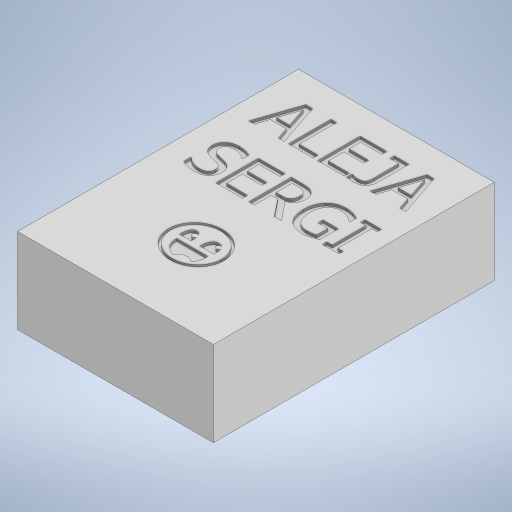
# Autodesk Inventor part: torta20personas
Saved by Autodesk Inventor 2024 (Build 280153000, 153)
## iProperties
Created: 2023-09-01
Part Number: torta20personas
Material: Genérico
Document SubType Name: Modeling
Designer: profe
Density: 1 g/cm^3
Appearance: Valor por defecto
Author: profe
Autodesk Inventor part; units mm, degrees
note: some values were not read from the file. Chosen so that the rebuilt part matches the saved one: offset side; direction of "Repujado1".
ref_plane "YZ Plane" through (0, 0, 0) normal (1, 0, 0) x (0, 1, 0)
ref_plane "XZ Plane" through (0, 0, 0) normal (0, 1, 0) x (-1, 0, 0)
ref_plane "XY Plane" through (0, 0, 0) normal (0, 0, 1) x (1, 0, 0)
sketch "Boceto2" plane through (0, 0, 0) normal (0, 1, 0) x (-1, 0, 0)
  line L0 (-115, -165) -> (115, -165)
  line L1 (115, -165) -> (115, 165)
  line L2 (115, 165) -> (-115, 165)
  line L3 (-115, 165) -> (-115, -165)
  line L4 (-115, -165) -> (115, 165) construction
  line L5 (115, -165) -> (-115, 165) construction
  point P0 (0, 0)
  dimension "d3" = 330
  dimension "d4" = 230
  constraints: 12 end point, 2 midpoint, 2 parallel, 1 horizontal, 1 perpendicular
  measures "d3" distance of L0.end L1.end
  measures "d4" distance of L0.start L0.end
extrude "Extrusión2" add sketch "Boceto2" along normal blind 100
sketch "Boceto3" plane through (0, 100, 0) normal (0, 1, 0) x (1, 0, 0)
  line L0 (-91.3257, 133.12) -> (-76.7106, 133.12) construction
  line L1 (-76.7106, 133.12) -> (-76.7106, 124.9893) construction
  line L2 (-76.7106, 124.9893) -> (-91.3257, 124.9893) construction
  line L3 (-91.3257, 124.9893) -> (-91.3257, 133.12) construction
  line L4 (-91.6498, 83.12) -> (-74.7941, 133.12)
  line L5 (-74.7941, 133.12) -> (-66.6093, 133.12)
  line L6 (-66.6093, 133.12) -> (-49.7536, 83.12)
  line L7 (-49.7536, 83.12) -> (-56.7633, 83.12)
  line L8 (-56.7633, 83.12) -> (-61.3014, 97.0989)
  line L9 (-61.3014, 97.0989) -> (-80.3857, 97.0989)
  line L10 (-80.3857, 97.0989) -> (-84.9237, 83.12)
  line L11 (-84.9237, 83.12) -> (-91.6498, 83.12)
  line L12 (-63.1247, 102.7716) -> (-70.8638, 126.3129)
  line L13 (-70.8638, 126.3129) -> (-78.5623, 102.7716)
  line L14 (-78.5623, 102.7716) -> (-63.1247, 102.7716)
  line L15 (-16.0421, 83.12) -> (-45.0129, 83.12)
  line L16 (-45.0129, 83.12) -> (-45.0129, 133.12)
  line L17 (-45.0129, 133.12) -> (-38.3678, 133.12)
  line L18 (-38.3678, 133.12) -> (-38.3678, 89.0357)
  line L19 (-38.3678, 89.0357) -> (-16.0421, 89.0357)
  line L20 (-16.0421, 89.0357) -> (-16.0421, 83.12)
  line L21 (-10.8152, 83.12) -> (-10.8152, 133.12)
  line L22 (-10.8152, 133.12) -> (20.4652, 133.12)
  line L23 (20.4652, 133.12) -> (20.4652, 127.2043)
  line L24 (20.4652, 127.2043) -> (-4.1701, 127.2043)
  line L25 (-4.1701, 127.2043) -> (-4.1701, 113.509)
  line L26 (-4.1701, 113.509) -> (18.804, 113.509)
  line L27 (18.804, 113.509) -> (18.804, 107.5933)
  line L28 (18.804, 107.5933) -> (-4.1701, 107.5933)
  line L29 (-4.1701, 107.5933) -> (-4.1701, 89.0357)
  line L30 (-4.1701, 89.0357) -> (20.4652, 89.0357)
  line L31 (20.4652, 89.0357) -> (20.4652, 83.12)
  line L32 (20.4652, 83.12) -> (-10.8152, 83.12)
  spline S0 degree 2 poles (46.5998, 96.1265) (46.5998, 89.5625) (38.5771, 82.4312) (31.8104, 82.4312) knots 0 0 0 1 2 2 2
  spline S1 degree 2 poles (31.8104, 82.4312) (30.1897, 82.4312) (24.8007, 82.9985) (22.9774, 83.4036) knots 0 0 0 1 2 2 2
  line L33 (22.9774, 83.4036) -> (22.9774, 89.8056)
  line L34 (22.9774, 89.8056) -> (23.3421, 89.8056)
  spline S2 degree 2 poles (23.3421, 89.8056) (24.7197, 89.3194) (28.8121, 88.1848) (30.919, 88.1848) knots 0 0 0 1 2 2 2
  spline S3 degree 2 poles (30.919, 88.1848) (33.9985, 88.1848) (37.6857, 89.603) (38.5365, 90.8996) knots 0 0 0 1 2 2 2
  spline S4 degree 2 poles (38.5365, 90.8996) (39.4685, 92.2367) (39.9547, 96.1265) (39.9547, 98.6792) knots 0 0 0 1 2 2 2
  line L35 (39.9547, 98.6792) -> (39.9547, 127.8121)
  line L36 (39.9547, 127.8121) -> (29.3793, 127.8121)
  line L37 (29.3793, 127.8121) -> (29.3793, 133.12)
  line L38 (29.3793, 133.12) -> (46.5998, 133.12)
  line L39 (46.5998, 133.12) -> (46.5998, 96.1265)
  line L40 (51.0163, 83.12) -> (67.872, 133.12)
  line L41 (67.872, 133.12) -> (76.0568, 133.12)
  line L42 (76.0568, 133.12) -> (92.9126, 83.12)
  line L43 (92.9126, 83.12) -> (85.9028, 83.12)
  line L44 (85.9028, 83.12) -> (81.3647, 97.0989)
  line L45 (81.3647, 97.0989) -> (62.2805, 97.0989)
  line L46 (62.2805, 97.0989) -> (57.7424, 83.12)
  line L47 (57.7424, 83.12) -> (51.0163, 83.12)
  line L48 (79.5414, 102.7716) -> (71.8023, 126.3129)
  line L49 (71.8023, 126.3129) -> (64.1038, 102.7716)
  line L50 (64.1038, 102.7716) -> (79.5414, 102.7716)
  spline S5 degree 2 poles (-72.3225, -0.0951) (-77.7519, -0.0951) (-85.3695, 2.174) (-88.7325, 3.7947) knots 0 0 0 1 2 2 2
  line L51 (-88.7325, 3.7947) -> (-88.7325, 12.1415)
  line L52 (-88.7325, 12.1415) -> (-88.2463, 12.1415)
  spline S6 degree 2 poles (-88.2463, 12.1415) (-84.9643, 9.0621) (-76.6579, 5.6586) (-72.8087, 5.6586) knots 0 0 0 1 2 2 2
  spline S7 degree 2 poles (-72.8087, 5.6586) (-67.2981, 5.6586) (-61.666, 10.2372) (-61.666, 14.0054) knots 0 0 0 1 2 2 2
  spline S8 degree 2 poles (-61.666, 14.0054) (-61.666, 17.0038) (-64.6239, 20.7315) (-67.8249, 21.6634) knots 0 0 0 1 2 2 2
  spline S9 degree 2 poles (-67.8249, 21.6634) (-70.1344, 22.3117) (-73.9837, 23.2031) (-76.8605, 23.9325) knots 0 0 0 1 2 2 2
  spline S10 degree 2 poles (-76.8605, 23.9325) (-79.4537, 24.6213) (-83.5461, 26.6877) (-85.1263, 28.349) knots 0 0 0 1 2 2 2
  spline S11 degree 2 poles (-85.1263, 28.349) (-86.666, 30.0103) (-88.3678, 34.4673) (-88.3678, 37.3847) knots 0 0 0 1 2 2 2
  spline S12 degree 2 poles (-88.3678, 37.3847) (-88.3678, 43.4625) (-78.8865, 51.6877) (-71.5526, 51.6877) knots 0 0 0 1 2 2 2
  spline S13 degree 2 poles (-71.5526, 51.6877) (-67.3387, 51.6877) (-59.8832, 50.0265) (-56.6823, 48.4462) knots 0 0 0 1 2 2 2
  line L53 (-56.6823, 48.4462) -> (-56.6823, 40.5046)
  line L54 (-56.6823, 40.5046) -> (-57.1685, 40.5046)
  spline S14 degree 2 poles (-57.1685, 40.5046) (-59.5591, 42.6926) (-67.0145, 45.9341) (-71.1069, 45.9341) knots 0 0 0 1 2 2 2
  spline S15 degree 2 poles (-71.1069, 45.9341) (-75.726, 45.9341) (-81.4391, 41.5986) (-81.4391, 38.0735) knots 0 0 0 1 2 2 2
  spline S16 degree 2 poles (-81.4391, 38.0735) (-81.4391, 34.913) (-78.0761, 31.1448) (-74.9156, 30.2939) knots 0 0 0 1 2 2 2
  spline S17 degree 2 poles (-74.9156, 30.2939) (-72.8087, 29.7266) (-66.6904, 28.268) (-64.6644, 27.6602) knots 0 0 0 1 2 2 2
  spline S18 degree 2 poles (-64.6644, 27.6602) (-59.5186, 26.08) (-54.7374, 19.7185) (-54.7374, 15.0589) knots 0 0 0 1 2 2 2
  spline S19 degree 2 poles (-54.7374, 15.0589) (-54.7374, 12.101) (-57.128, 6.4284) (-59.2754, 4.443) knots 0 0 0 1 2 2 2
  spline S20 degree 2 poles (-59.2754, 4.443) (-61.666, 2.255) (-67.7438, -0.0951) (-72.3225, -0.0951) knots 0 0 0 1 2 2 2
  line L55 (-47.9707, 0.7963) -> (-47.9707, 50.7963)
  line L56 (-47.9707, 50.7963) -> (-16.6904, 50.7963)
  line L57 (-16.6904, 50.7963) -> (-16.6904, 44.8806)
  line L58 (-16.6904, 44.8806) -> (-41.3257, 44.8806)
  line L59 (-41.3257, 44.8806) -> (-41.3257, 31.1853)
  line L60 (-41.3257, 31.1853) -> (-18.3516, 31.1853)
  line L61 (-18.3516, 31.1853) -> (-18.3516, 25.2696)
  line L62 (-18.3516, 25.2696) -> (-41.3257, 25.2696)
  line L63 (-41.3257, 25.2696) -> (-41.3257, 6.712)
  line L64 (-41.3257, 6.712) -> (-16.6904, 6.712)
  line L65 (-16.6904, 6.712) -> (-16.6904, 0.7963)
  line L66 (-16.6904, 0.7963) -> (-47.9707, 0.7963)
  line L67 (29.2983, 0.7963) -> (20.6678, 0.7963)
  line L68 (20.6678, 0.7963) -> (4.8656, 20.691)
  line L69 (4.8656, 20.691) -> (-2.7519, 20.691)
  line L70 (-2.7519, 20.691) -> (-2.7519, 0.7963)
  line L71 (-2.7519, 0.7963) -> (-9.397, 0.7963)
  line L72 (-9.397, 0.7963) -> (-9.397, 50.7963)
  line L73 (-9.397, 50.7963) -> (3.4879, 50.7963)
  spline S21 degree 2 poles (3.4879, 50.7963) (7.7829, 50.7963) (13.5771, 49.8644) (16.2108, 48.1626) knots 0 0 0 1 2 2 2
  spline S22 degree 2 poles (16.2108, 48.1626) (18.8445, 46.4608) (21.8834, 41.1529) (21.8834, 37.2226) knots 0 0 0 1 2 2 2
  spline S23 degree 2 poles (21.8834, 37.2226) (21.8834, 31.7526) (16.2918, 24.3377) (11.5106, 22.5548) knots 0 0 0 1 2 2 2
  line L74 (11.5106, 22.5548) -> (29.2983, 0.7963)
  spline S24 degree 2 poles (14.9547, 36.6958) (14.9547, 38.8838) (13.415, 42.2469) (11.7942, 43.3409) knots 0 0 0 1 2 2 2
  spline S25 degree 2 poles (11.7942, 43.3409) (10.3761, 44.2728) (6.6079, 45.0427) (3.8526, 45.0427) knots 0 0 0 1 2 2 2
  line L75 (3.8526, 45.0427) -> (-2.7519, 45.0427)
  line L76 (-2.7519, 45.0427) -> (-2.7519, 26.242)
  line L77 (-2.7519, 26.242) -> (3.0827, 26.242)
  spline S26 degree 2 poles (3.0827, 26.242) (5.9596, 26.242) (10.5382, 27.255) (12.1184, 28.8352) knots 0 0 0 1 2 2 2
  spline S27 degree 2 poles (12.1184, 28.8352) (13.5771, 30.2129) (14.9547, 34.1026) (14.9547, 36.6958) knots 0 0 0 1 2 2 2
  spline S28 degree 2 poles (54.2173, -0.1761) (48.9093, -0.1761) (40.1168, 3.0654) (36.9563, 6.3474) knots 0 0 0 1 2 2 2
  spline S29 degree 2 poles (36.9563, 6.3474) (33.7959, 9.6699) (30.4328, 19.4754) (30.4328, 25.8368) knots 0 0 0 1 2 2 2
  spline S30 degree 2 poles (30.4328, 25.8368) (30.4328, 31.8741) (33.8364, 41.4365) (36.9968, 44.8401) knots 0 0 0 1 2 2 2
  spline S31 degree 2 poles (36.9968, 44.8401) (40.0357, 48.1221) (48.9498, 51.6877) (54.2578, 51.6877) knots 0 0 0 1 2 2 2
  spline S32 degree 2 poles (54.2578, 51.6877) (56.8104, 51.6877) (61.4296, 50.9584) (63.5365, 50.3101) knots 0 0 0 1 2 2 2
  spline S33 degree 2 poles (63.5365, 50.3101) (65.2383, 49.8239) (69.3712, 48.0411) (70.6273, 47.3928) knots 0 0 0 1 2 2 2
  line L78 (70.6273, 47.3928) -> (70.6273, 39.3701)
  line L79 (70.6273, 39.3701) -> (70.06, 39.3701)
  spline S34 degree 2 poles (70.06, 39.3701) (68.804, 40.4641) (66.1703, 42.4495) (63.7391, 43.584) knots 0 0 0 1 2 2 2
  spline S35 degree 2 poles (63.7391, 43.584) (61.7132, 44.597) (56.4863, 45.9341) (53.4879, 45.9341) knots 0 0 0 1 2 2 2
  spline S36 degree 2 poles (53.4879, 45.9341) (46.2756, 45.9341) (37.3615, 35.0751) (37.3615, 26.0394) knots 0 0 0 1 2 2 2
  spline S37 degree 2 poles (37.3615, 26.0394) (37.3615, 21.0151) (39.7116, 13.4787) (41.9401, 10.8855) knots 0 0 0 1 2 2 2
  spline S38 degree 2 poles (41.9401, 10.8855) (44.0876, 8.2923) (50.1654, 5.5775) (53.9741, 5.5775) knots 0 0 0 1 2 2 2
  spline S39 degree 2 poles (53.9741, 5.5775) (56.7699, 5.5775) (62.3615, 6.3879) (64.2659, 7.1983) knots 0 0 0 1 2 2 2
  line L80 (64.2659, 7.1983) -> (64.2659, 20.1237)
  line L81 (64.2659, 20.1237) -> (52.6775, 20.1237)
  line L82 (52.6775, 20.1237) -> (52.6775, 25.9584)
  line L83 (52.6775, 25.9584) -> (70.8299, 25.9584)
  line L84 (70.8299, 25.9584) -> (70.8299, 4.1189)
  spline S40 degree 2 poles (70.8299, 4.1189) (69.5738, 3.5516) (65.2788, 1.8093) (63.4555, 1.2826) knots 0 0 0 1 2 2 2
  spline S41 degree 2 poles (63.4555, 1.2826) (60.9839, 0.5532) (57.013, -0.1761) (54.2173, -0.1761) knots 0 0 0 1 2 2 2
  line L85 (96.5998, 0.7963) -> (77.2318, 0.7963)
  line L86 (77.2318, 0.7963) -> (77.2318, 5.9017)
  line L87 (77.2318, 5.9017) -> (83.5933, 5.9017)
  line L88 (83.5933, 5.9017) -> (83.5933, 45.691)
  line L89 (83.5933, 45.691) -> (77.2318, 45.691)
  line L90 (77.2318, 45.691) -> (77.2318, 50.7963)
  line L91 (77.2318, 50.7963) -> (96.5998, 50.7963)
  line L92 (96.5998, 50.7963) -> (96.5998, 45.691)
  line L93 (96.5998, 45.691) -> (90.2383, 45.691)
  line L94 (90.2383, 45.691) -> (90.2383, 5.9017)
  line L95 (90.2383, 5.9017) -> (96.5998, 5.9017)
  line L96 (96.5998, 5.9017) -> (96.5998, 0.7963)
  point P0 (0, 0)
  constraints: 2 other
sketch "Boceto4" plane through (0, 100, 0) normal (0, 1, 0) x (1, 0, 0)
  ellipse E0 centre (3.3562, -73.5305) end of major axis (35.95, -73.5305) minor radius 30.9478
  line L0 (-17.1173, -72.8754) -> (-3.3591, -72.8754)
  line L1 (-3.3591, -72.8754) -> (-3.3591, -65.0877) construction
  line L2 (-3.3591, -65.0877) -> (-6.2828, -57.898) construction
  line L3 (-6.2828, -57.898) -> (-11.4475, -57.898) construction
  line L4 (-11.4475, -57.898) -> (-17.1173, -61.4929) construction
  line L5 (-17.1173, -61.4929) -> (-17.1173, -72.8754) construction
  spline S0 degree 4 poles (-3.3591, -72.8754) (-3.3591, -65.0877) (-6.2828, -57.898) (-11.4475, -57.898) (-17.1173, -61.4929) (-17.1173, -72.8754) knots 1 1 1 1 1 2 3 3 3 3 3
  line L6 (6.7957, -72.8754) -> (23.6015, -72.8754)
  line L7 (23.6015, -72.8754) -> (23.6015, -65.0877) construction
  line L8 (23.6015, -65.0877) -> (20.2264, -57.898) construction
  line L9 (20.2264, -57.898) -> (16.8082, -57.898) construction
  line L10 (16.8082, -57.898) -> (6.7957, -59.6954) construction
  line L11 (6.7957, -59.6954) -> (6.7957, -72.8754) construction
  spline S1 degree 4 poles (23.6015, -72.8754) (23.6015, -65.0877) (20.2264, -57.898) (16.8082, -57.898) (6.7957, -59.6954) (6.7957, -72.8754) knots 1 1 1 1 1 2 3 3 3 3 3
  line L12 (21.9139, -78.608) -> (-14.5441, -78.608)
  line L13 (21.9139, -78.608) -> (23.6015, -89.9597) construction
  line L14 (23.6015, -89.9597) -> (13.551, -97.3256) construction
  line L15 (13.551, -97.3256) -> (3.6849, -101.6803) construction
  line L16 (3.6849, -101.6803) -> (-10.2382, -93.6427) construction
  line L17 (-10.2382, -93.6427) -> (-14.5441, -86.0791) construction
  line L18 (-14.5441, -86.0791) -> (-14.5441, -78.608) construction
  spline S2 degree 4 poles (21.9139, -78.608) (23.6015, -89.9597) (13.551, -97.3256) (3.6849, -101.6803) (-10.2382, -93.6427) (-14.5441, -86.0791) (-14.5441, -78.608) knots 1 1 1 1 1 2 3 4 4 4 4 4
  line L19 (-0.0545, -97.6615) -> (3.6849, -91.2682) construction
  line L20 (3.6849, -91.2682) -> (8.618, -89.8609) construction
  line L21 (8.618, -89.8609) -> (12.2197, -89.8609) construction
  line L22 (12.2197, -89.8609) -> (17.4754, -93.6427) construction
  spline S3 degree 4 poles (-0.0545, -97.6615) (3.6849, -91.2682) (8.618, -89.8609) (12.2197, -89.8609) (17.4754, -93.6427) knots 1 1 1 1 1 2 2 2 2 2
  arc A0 (-5.217, -62.3766) -> (-3.8659, -66.4524) centre (-6.5721, -65.0877) ccw
  arc A1 (20.015, -60.2235) -> (22.3703, -63.936) centre (19.6064, -63.0861) ccw
  spline S4 degree 5 poles (33.1537, -73.5305) (33.1534, -69.0757) (32.2217, -64.6175) (30.351, -60.4297) (24.9525, -52.8953) (17.0938, -47.9476) (12.6537, -46.2366) (3.3562, -44.5213) (-5.9413, -46.2367) (-10.3815, -47.9473) (-18.24, -52.8959) (-23.6388, -60.429) (-25.509, -64.6191) (-27.3736, -73.5305) (-25.509, -82.442) (-23.6388, -86.6321) (-18.24, -94.1651) (-10.3815, -99.1138) (-5.9413, -100.8243) (3.3562, -102.5398) (12.6537, -100.8245) (17.0938, -99.1135) (24.9525, -94.1658) (30.351, -86.6313) (32.2217, -82.4436) (33.1534, -77.9853) (33.1537, -73.5305) knots 0 0 0 0 0 0 0.122343 0.122343 0.122343 0.25 0.25 0.25 0.377657 0.377657 0.377657 0.5 0.5 0.5 0.622343 0.622343 0.622343 0.75 0.75 0.75 0.877657 0.877657 0.877657 1 1 1 1 1 1
  point P0 (0, 0)
  constraints: 6 end point, 6 horizontal, 4 point on circle, 3 centre point, 2 vertical, 21 other
extrude "Extrusión3" cut sketch "Boceto4" against normal blind 3 contours E0 | S0 A0 L0 | S1 A1 L6 | S2 S3 L12
emboss "Repujado1" sketch "Boceto3" operation cut depth 3 direction (0, -1, 0)
